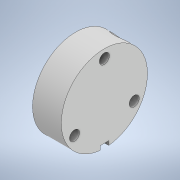
# Autodesk Inventor part: 711124
Saved by Autodesk Inventor 2022 (Build 260153000, 153)
## iProperties
Created: 2021-10-21
Part Number: 711124
Material: Типовые
Document SubType Name: Modeling
Designer: RaNSiD
Density: 1 g/cm^3
Appearance: По умолчанию
Author: RaNSiD
Autodesk Inventor part; units mm, degrees
ref_plane "YZ Plane" through (0, 0, 0) normal (1, 0, 0) x (0, 1, 0)
ref_plane "XZ Plane" through (0, 0, 0) normal (0, 1, 0) x (-1, 0, 0)
sketch "Эскиз1" plane through (0, 0, 0) normal (0, 0, 1) x (1, 0, 0)
  line L0 (0, 0) -> (20, 0)
  line L1 (20, 0) -> (20, 30)
  line L2 (20, 30) -> (0, 30)
  line L3 (0, 30) -> (0, 0)
  dimension "d0" = 20
  dimension "d1" = 30
  constraints: 8 end point, 2 parallel, 1 horizontal, 1 perpendicular
  measures "d0" distance of L2.end L1.end
  measures "d1" distance of L1.end L0.end
revolve "Вращение1" add sketch "Эскиз1" angle 360 about axis through (0, 0, 0) along (1, 0, 0)
sketch "Эскиз2" plane through (0, 0, 0) normal (-1, 0, 0) x (0, 0, 1)
  point P0 (0, 0)
  point P1 (0, 24)
  point P2 (-20.7846, -12)
  point P3 (20.7846, -12)
  dimension "d3" = 24
  dimension "d6" = 360
  constraints: 4 other
  measures "d3" distance of point (0, 0) point (0, 24)
hole "Отверстие1" at (0, 24, 0) at (0, -12, -20.7846) at (0, -12, 20.7846) direction (1, 0, 0) diameter 7 end through all counterbore diameter 9 counterbore depth 5
sketch "Эскиз3" plane through (0, 0, 0) normal (-1, 0, 0) x (0, 0, 1)
  point P0 (0, 0)
  point P1 (0, 0)
  constraints: 1 coincident
hole "Отверстие2" at (0, 0, 0) direction (1, 0, 0) diameter 30 depth 16 countersink diameter 34 countersink angle 90
sketch "Эскиз4" plane through (0, 0, 0) normal (-1, 0, 0) x (0, 0, 1)
  circle A0 centre (0, 0) radius 30 construction
  line L0 (-3, -27) -> (3, -27)
  line L1 (3, -27) -> (3, -29.8496)
  line L2 (-3, -29.8496) -> (-3, -27)
  arc A1 (-3, -29.8496) -> (3, -29.8496) centre (0, 0) ccw
  point P0 (0, -27)
  dimension "d22" = 6
  dimension "d23" = 27
  constraints: 6 end point, 4 point on circle, 1 centre point, 1 concentric, 1 horizontal, 1 midpoint, 1 parallel, 1 perpendicular, 1 vertical alignment
  measures "d22" distance of L0.start L0.end
  measures "d23" distance of point (0, -27) point (0, 0)
extrude "Выдавливание1" cut sketch "Эскиз4" against normal blind 20
ref_plane "РабПлоскость1" through (10, -29.8496, -3) normal (-1, 0, 0) x (0, 0, 1)
sketch "Эскиз5" plane through (10, -29.8496, -3) normal (-1, 0, 0) x (0, 0, 1)
  line L0 (3, 29.8496) -> (-21.7487, 54.5984) construction
  line L1 (3, 29.8496) -> (33, 29.8496) construction
  arc A0 (6, 0) -> (0, 0) centre (3, 29.8496) ccw construction
  circle A1 centre (3, 29.8496) radius 15 construction
  arc A2 (-6.0161, 41.8375) -> (-8.9879, 38.8657) centre (3, 29.8496) ccw
  line L2 (-7.6066, 40.4562) -> (-21.7487, 54.5984)
  line L3 (-6.0161, 41.8375) -> (-16.4454, 59.9017)
  line L4 (-8.9879, 38.8657) -> (-27.052, 49.2951)
  line L5 (-27.052, 49.2951) -> (-16.4454, 59.9017)
  dimension "d27" = 135
  dimension "d32" = 15
  dimension "d33" = 15
  dimension "d34" = 20
  dimension "d35" = 15
  constraints: 12 end point, 6 point on circle, 1 centre point, 1 coincident, 1 collinear, 1 equal length, 1 horizontal, 1 midpoint, 1 point on line
  measures "d27" angle of L1 L0
  measures "d32" angle of L0 L3
  measures "d33" angle of L4 L0
  measures "d34" distance of L2.start L0.end
  measures "d35" distance of L4.end L3.end
revolve "Вращение3" cut sketch "Эскиз5" angle 360 about axis through (10, 0, 0) along (0, 0.7071068, -0.7071068) contours A2 L2 L5 L3
